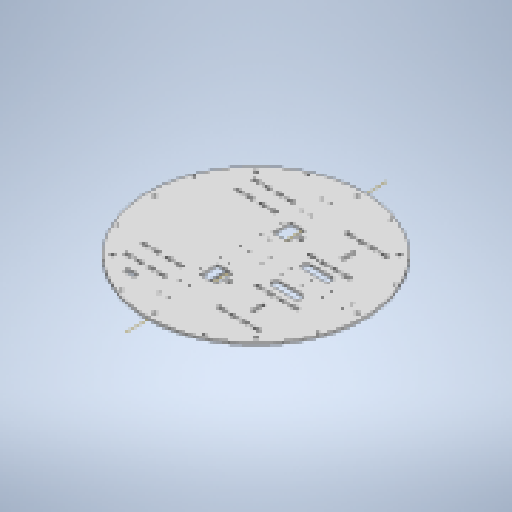
# Autodesk Inventor part: Osn. platform
Saved by Autodesk Inventor 2023.1 (Build 271208000, 208)
## iProperties
Created: 2023-03-13
Part Number: Osn. platform
Material: Типовые
Document SubType Name: Modeling
Designer: User
Density: 1 g/cm^3
Appearance: По умолчанию
Mass: 865.132 g
Surface Area: 3668.91 cm^2
Volume: 865.132 cm^3
Author: User
Autodesk Inventor part; units mm, degrees
ref_plane "YZ Plane" through (0, 0, 0) normal (1, 0, 0) x (0, 1, 0)
ref_plane "XZ Plane" through (0, 0, 0) normal (0, 1, 0) x (-1, 0, 0)
ref_plane "XY Plane" through (0, 0, 0) normal (0, 0, 1) x (1, 0, 0)
sketch "Основ. платформа" plane through (0, 0, 0) normal (0, 1, 0) x (-1, 0, 0)
  circle A0 centre (0, 0) radius 240
  line L0 (160.351, 321.3144) -> (160.351, -249.4153)
  point P0 (160.351, -178.5709)
  point P1 (160.351, 178.5709)
  dimension "d117" = 480
  constraints: 2 end point, 1 centre point, 1 coincident, 1 vertical
  measures "d117" diameter of A0
extrude "Осн. платформа" add sketch "Основ. платформа" along normal blind 5 contours L0 A0 picked at (27.6333, -10.8021)
sketch "Эскиз14" plane through (0, 5, 0) normal (0, 1, 0) x (0, 0, -1)
  line L0 (111.049, 144.9298) -> (124.3347, 144.9298)
  line L1 (124.3347, 144.9298) -> (124.3347, 138.9298)
  line L2 (111.049, 138.9298) -> (124.3347, 138.9298)
  line L3 (111.049, 144.9298) -> (111.049, 138.9298)
  line L4 (137.6204, 144.9298) -> (150.9061, 144.9298)
  line L5 (150.9061, 144.9298) -> (150.9061, 138.9298)
  line L6 (137.6204, 138.9298) -> (150.9061, 138.9298)
  line L7 (137.6204, 144.9298) -> (137.6204, 138.9298)
  line L8 (137.6204, 138.9298) -> (124.3347, 144.9298) construction
  line L9 (111.049, -61.9298) -> (124.3347, -61.9298)
  line L10 (111.049, -61.9298) -> (111.049, -55.9298)
  line L11 (97.7633, -61.9298) -> (97.7633, -55.9298)
  line L12 (71.1919, -61.9298) -> (71.1919, -55.9298)
  line L13 (57.9061, -61.9298) -> (57.9061, -55.9298)
  line L14 (57.9061, -55.9298) -> (71.1919, -55.9298)
  line L15 (57.9061, -61.9298) -> (71.1919, -61.9298)
  line L16 (107.4061, -87.5965) -> (101.4061, -87.5965)
  line L17 (101.4061, -87.5965) -> (101.4061, -113.2631)
  line L18 (107.4061, -113.2631) -> (107.4061, -87.5965)
  line L19 (57.9061, -138.9298) -> (71.1919, -138.9298)
  line L20 (101.4061, -113.2631) -> (107.4061, -113.2631)
  line L21 (84.4776, -138.9298) -> (97.7633, -138.9298)
  line L22 (84.4776, -144.9298) -> (84.4776, -138.9298)
  line L23 (84.4776, -144.9298) -> (97.7633, -144.9298)
  line L24 (97.7633, -144.9298) -> (97.7633, -138.9298)
  line L25 (111.049, -144.9298) -> (111.049, -138.9298)
  line L26 (111.049, -138.9298) -> (124.3347, -138.9298)
  line L27 (111.049, -144.9298) -> (124.3347, -144.9298)
  line L28 (124.3347, -144.9298) -> (124.3347, -138.9298)
  line L29 (137.6204, -61.9298) -> (150.9061, -61.9298)
  line L30 (150.9061, -61.9298) -> (150.9061, -55.9298)
  line L31 (137.6204, -55.9298) -> (150.9061, -55.9298)
  line L32 (137.6204, -61.9298) -> (137.6204, -55.9298)
  circle A0 centre (130.9776, -58.9298) radius 1.5
  line L33 (137.6204, -144.9298) -> (137.6204, -138.9298)
  line L34 (137.6204, -144.9298) -> (150.9061, -144.9298)
  line L35 (150.9061, -144.9298) -> (150.9061, -138.9298)
  line L36 (137.6204, -138.9298) -> (150.9061, -138.9298)
  line L37 (124.3347, -61.9298) -> (124.3347, -55.9298)
  line L38 (111.049, -55.9298) -> (124.3347, -55.9298)
  line L39 (84.4776, -61.9298) -> (97.7633, -61.9298)
  line L40 (84.4776, -55.9298) -> (97.7633, -55.9298)
  line L41 (84.4776, -61.9298) -> (84.4776, -55.9298)
  line L42 (71.1919, -144.9298) -> (71.1919, -138.9298)
  line L43 (57.9061, -144.9298) -> (71.1919, -144.9298)
  line L44 (57.9061, -144.9298) -> (57.9061, -138.9298)
  circle A1 centre (77.5336, -58.9298) radius 1.5
  circle A2 centre (130.9776, -141.9298) radius 1.5
  line L45 (137.6204, -138.9298) -> (124.3347, -144.9298) construction
  circle A3 centre (104.2556, -141.9298) radius 1.5
  circle A4 centre (77.5336, -141.9298) radius 1.5
  circle A5 centre (104.2556, -58.9298) radius 1.5
  line L46 (0, 238.0276) -> (0, -238.2088) construction
  line L47 (-70.7885, 145.0999) -> (-57.9314, 145.0999)
  line L48 (-57.9314, 145.0999) -> (-57.9314, 139.0999)
  line L49 (-57.9314, 139.0999) -> (-70.7885, 139.0999)
  line L50 (-70.7885, 139.0999) -> (-70.7885, 145.0999)
  line L51 (-70.7885, 106.8999) -> (-57.9314, 106.8999)
  line L52 (-57.9314, 106.8999) -> (-57.9314, 100.8999)
  line L53 (-57.9314, 100.8999) -> (-70.7885, 100.8999)
  line L54 (-70.7885, 100.8999) -> (-70.7885, 106.8999)
  line L55 (-70.7885, 145.0999) -> (-70.7885, 156.3999) construction
  line L56 (-70.7885, 100.8999) -> (-70.7885, 89.5999) construction
  line L57 (-96.5028, 100.8999) -> (-96.5028, 106.8999)
  line L58 (-96.5028, 106.8999) -> (-83.6457, 106.8999)
  line L59 (-83.6457, 139.0999) -> (-96.5028, 139.0999)
  line L60 (-83.6457, 100.8999) -> (-96.5028, 100.8999)
  line L61 (-83.6457, 145.0999) -> (-83.6457, 139.0999)
  line L62 (-96.5028, 139.0999) -> (-96.5028, 145.0999)
  line L63 (-96.5028, 145.0999) -> (-83.6457, 145.0999)
  line L64 (-83.6457, 106.8999) -> (-83.6457, 100.8999)
  line L65 (-122.2171, 100.8999) -> (-122.2171, 106.8999)
  line L66 (-122.2171, 106.8999) -> (-109.36, 106.8999)
  line L67 (-109.36, 139.0999) -> (-122.2171, 139.0999)
  line L68 (-109.36, 100.8999) -> (-122.2171, 100.8999)
  line L69 (-109.36, 145.0999) -> (-109.36, 139.0999)
  line L70 (-122.2171, 139.0999) -> (-122.2171, 145.0999)
  line L71 (-122.2171, 145.0999) -> (-109.36, 145.0999)
  line L72 (-109.36, 106.8999) -> (-109.36, 100.8999)
  line L73 (-147.9314, 100.8999) -> (-147.9314, 106.8999)
  line L74 (-147.9314, 106.8999) -> (-135.0743, 106.8999)
  line L75 (-135.0743, 139.0999) -> (-147.9314, 139.0999)
  line L76 (-135.0743, 100.8999) -> (-147.9314, 100.8999)
  line L77 (-135.0743, 145.0999) -> (-135.0743, 139.0999)
  line L78 (-147.9314, 139.0999) -> (-147.9314, 145.0999)
  line L79 (-147.9314, 145.0999) -> (-135.0743, 145.0999)
  line L80 (-135.0743, 106.8999) -> (-135.0743, 100.8999)
  line L81 (-135.0743, 139.0999) -> (-122.2171, 145.0999) construction
  line L82 (-83.6457, 139.0999) -> (-70.7885, 145.0999) construction
  line L83 (-135.0743, 100.8999) -> (-122.2171, 106.8999) construction
  line L84 (-83.6457, 100.8999) -> (-70.7885, 106.8999) construction
  circle A6 centre (-128.6457, 142.0999) radius 1.5
  circle A7 centre (-77.2171, 142.0999) radius 1.5
  circle A8 centre (-77.2171, 103.8999) radius 1.5
  circle A9 centre (-128.6457, 103.8999) radius 1.5
  line L85 (-147.9314, 145.0999) -> (-147.9314, 139.0999) projected
  line L86 (-135.0743, 145.0999) -> (-147.9314, 145.0999) projected
  arc A10 (-178.5709, 160.351) -> (178.5709, 160.351) centre (0, 0) ccw projected
  line L87 (-240, 0) -> (0, 0) construction
  line L88 (-122.2171, -139.0999) -> (-122.2171, -145.0999)
  line L89 (-147.9314, -145.0999) -> (-135.0743, -145.0999)
  line L90 (-147.9314, -139.0999) -> (-147.9314, -145.0999)
  line L91 (-96.5028, -106.8999) -> (-83.6457, -106.8999)
  line L92 (-96.5028, -100.8999) -> (-96.5028, -106.8999)
  line L93 (-83.6457, -100.8999) -> (-96.5028, -100.8999)
  line L94 (-83.6457, -106.8999) -> (-83.6457, -100.8999)
  line L95 (-83.6457, -100.8999) -> (-70.7885, -106.8999) construction
  circle A11 centre (-77.2171, -103.8999) radius 1.5
  line L96 (-70.7885, -100.8999) -> (-70.7885, -106.8999)
  line L97 (-70.7885, -106.8999) -> (-57.9314, -106.8999)
  line L98 (-57.9314, -106.8999) -> (-57.9314, -100.8999)
  line L99 (-57.9314, -100.8999) -> (-70.7885, -100.8999)
  line L100 (-70.7885, -100.8999) -> (-70.7885, -89.5999) construction
  line L101 (-122.2171, -100.8999) -> (-122.2171, -106.8999)
  line L102 (-147.9314, -100.8999) -> (-147.9314, -106.8999)
  line L103 (-135.0743, -145.0999) -> (-135.0743, -139.0999)
  line L104 (-135.0743, -139.0999) -> (-147.9314, -139.0999)
  line L105 (-147.9314, -106.8999) -> (-135.0743, -106.8999)
  line L106 (-135.0743, -106.8999) -> (-135.0743, -100.8999)
  line L107 (-135.0743, -100.8999) -> (-147.9314, -100.8999)
  line L108 (-109.36, -106.8999) -> (-109.36, -100.8999)
  line L109 (-109.36, -100.8999) -> (-122.2171, -100.8999)
  line L110 (-122.2171, -145.0999) -> (-109.36, -145.0999)
  line L111 (-122.2171, -106.8999) -> (-109.36, -106.8999)
  line L112 (-109.36, -139.0999) -> (-122.2171, -139.0999)
  circle A12 centre (-128.6457, -142.0999) radius 1.5
  circle A13 centre (-128.6457, -103.8999) radius 1.5
  line L113 (-135.0743, -100.8999) -> (-122.2171, -106.8999) construction
  line L114 (-109.36, -145.0999) -> (-109.36, -139.0999)
  line L115 (-135.0743, -139.0999) -> (-122.2171, -145.0999) construction
  line L116 (-70.7885, -145.0999) -> (-57.9314, -145.0999)
  line L117 (-57.9314, -145.0999) -> (-57.9314, -139.0999)
  line L118 (-57.9314, -139.0999) -> (-70.7885, -139.0999)
  line L119 (-70.7885, -139.0999) -> (-70.7885, -145.0999)
  circle A14 centre (-77.2171, -142.0999) radius 1.5
  line L120 (-83.6457, -139.0999) -> (-70.7885, -145.0999) construction
  line L121 (-83.6457, -145.0999) -> (-83.6457, -139.0999)
  line L122 (-70.7885, -145.0999) -> (-70.7885, -156.3999) construction
  line L123 (-96.5028, -145.0999) -> (-83.6457, -145.0999)
  line L124 (-96.5028, -139.0999) -> (-96.5028, -145.0999)
  line L125 (-83.6457, -139.0999) -> (-96.5028, -139.0999)
  line L126 (-147.9314, -145.0999) -> (-147.9314, -139.0999)
  line L127 (-135.0743, -145.0999) -> (-147.9314, -145.0999)
  line L128 (137.6204, 0) -> (-122.2171, 0) construction
  line L129 (97.7633, 61.9298) -> (97.7633, 55.9298)
  line L130 (84.4776, 55.9298) -> (97.7633, 55.9298)
  line L131 (84.4776, 61.9298) -> (84.4776, 55.9298)
  circle A15 centre (77.5336, 58.9298) radius 1.5
  line L132 (84.4776, 61.9298) -> (97.7633, 61.9298)
  circle A16 centre (104.2556, 58.9298) radius 1.5
  line L133 (111.049, 61.9298) -> (111.049, 55.9298)
  line L134 (111.049, 55.9298) -> (124.3347, 55.9298)
  line L135 (111.049, 61.9298) -> (124.3347, 61.9298)
  line L136 (124.3347, 61.9298) -> (124.3347, 55.9298)
  circle A17 centre (130.9776, 58.9298) radius 1.5
  line L137 (111.049, 138.9298) -> (124.3347, 138.9298)
  line L138 (111.049, 144.9298) -> (124.3347, 144.9298)
  line L139 (124.3347, 144.9298) -> (124.3347, 138.9298)
  circle A18 centre (130.9776, 141.9298) radius 1.5
  line L140 (137.6204, 138.9298) -> (124.3347, 144.9298) construction
  line L141 (137.6204, 144.9298) -> (137.6204, 138.9298)
  line L142 (137.6204, 138.9298) -> (150.9061, 138.9298)
  line L143 (137.6204, 144.9298) -> (150.9061, 144.9298)
  line L144 (150.9061, 144.9298) -> (150.9061, 138.9298)
  line L145 (137.6204, 61.9298) -> (137.6204, 55.9298)
  line L146 (137.6204, 55.9298) -> (150.9061, 55.9298)
  line L147 (137.6204, 61.9298) -> (150.9061, 61.9298)
  line L148 (150.9061, 61.9298) -> (150.9061, 55.9298)
  line L149 (107.4061, 87.5965) -> (101.4061, 87.5965)
  line L150 (101.4061, 87.5965) -> (101.4061, 113.2631)
  line L151 (107.4061, 113.2631) -> (107.4061, 87.5965)
  line L152 (111.049, 144.9298) -> (111.049, 138.9298)
  circle A19 centre (104.2556, 141.9298) radius 1.5
  line L153 (101.4061, 113.2631) -> (107.4061, 113.2631)
  line L154 (97.7633, 144.9298) -> (97.7633, 138.9298)
  line L155 (84.4776, 144.9298) -> (97.7633, 144.9298)
  line L156 (84.4776, 138.9298) -> (97.7633, 138.9298)
  line L157 (84.4776, 144.9298) -> (84.4776, 138.9298)
  circle A20 centre (77.5336, 141.9298) radius 1.5
  line L158 (71.1919, 61.9298) -> (71.1919, 55.9298)
  line L159 (57.9061, 144.9298) -> (57.9061, 138.9298)
  line L160 (57.9061, 144.9298) -> (71.1919, 144.9298)
  line L161 (71.1919, 144.9298) -> (71.1919, 138.9298)
  line L162 (57.9061, 138.9298) -> (71.1919, 138.9298)
  line L163 (57.9061, 61.9298) -> (57.9061, 55.9298)
  line L164 (57.9061, 61.9298) -> (71.1919, 61.9298)
  line L165 (57.9061, 55.9298) -> (71.1919, 55.9298)
  line L166 (11.3275, -97.2298) -> (11.3275, -64.2298) projected
  circle A21 centre (21.3275, -80.7298) radius 5.5
  circle A22 centre (19.3709, 80.7298) radius 5.5
  line L167 (9.3709, 64.2298) -> (9.3709, 97.2298) projected
  line L168 (11.3275, -80.7298) -> (40.4372, -80.7298)
  line L169 (9.3709, 80.7298) -> (30.4216, 80.7298)
  point P0 (-147.9314, -145.0886)
  point P1 (-147.9314, -145.0999)
  point P2 (-147.9108, -145.0999)
  point P3 (-135.0743, -145.0999)
  point P4 (-135.0743, 145.0999)
  point P5 (-147.9108, 145.0999)
  point P6 (-147.9314, 145.0999)
  point P7 (-147.9314, 145.0886)
  point P8 (-147.9314, 145.0999)
  dimension "d205" = 12.8571
  dimension "d206" = 6
  dimension "d207" = 25.7143
  dimension "d208" = 3
  dimension "d299" = 11
  dimension "d300" = 11
  dimension "d301" = 10
  dimension "d302" = 10
  constraints: 332 end point, 83 symmetric about line, 22 centre point, 8 equal length, 6 midpoint, 5 horizontal, 5 point on line, 3 equal radius, 2 collinear, 2 perpendicular, 2 vertical alignment, 1 point on circle, 1 vertical, 10 other
  measures "d205" distance of L48.end L49.end
  measures "d206" distance of L49.end L47.start
  measures "d207" distance of L54.start L57.start
  measures "d208" diameter of A9
  measures "d299" diameter of A21
  measures "d300" diameter of A22
  measures "d301" distance from line of L166 A21.centre
  measures "d302" distance from line of L167 A22.centre
extrude "Выдавливание9" cut sketch "Эскиз14" against normal up to surface (5 mm away)
sketch "Эскиз16" plane through (0, 5, 0) normal (0, 1, 0) x (0, 0, -1)
  line L0 (66.5859, 0) -> (-61.9521, 0) construction
  circle A0 centre (104.2556, -58.9298) radius 1.5 construction
  circle A1 centre (130.9776, -58.9298) radius 1.5 construction
  line L1 (125.6303, -33.4298) -> (77.5364, -33.4298) construction
  line L2 (125.6303, -24.4298) -> (77.5364, -24.4298)
  line L3 (77.5364, -42.4298) -> (125.6303, -42.4298)
  arc A2 (125.6303, -42.4298) -> (125.6303, -24.4298) centre (125.6303, -33.4298) ccw
  arc A3 (77.5364, -24.4298) -> (77.5364, -42.4298) centre (77.5364, -33.4298) ccw
  line L4 (125.6303, 33.4298) -> (77.5364, 33.4298) construction
  line L5 (125.6303, 24.4298) -> (77.5364, 24.4298)
  line L6 (77.5364, 42.4298) -> (125.6303, 42.4298)
  arc A4 (125.6303, 24.4298) -> (125.6303, 42.4298) centre (125.6303, 33.4298) ccw
  arc A5 (77.5364, 42.4298) -> (77.5364, 24.4298) centre (77.5364, 33.4298) ccw
  circle A6 centre (-225.3213, 0) radius 4
  circle A7 centre (-159.3262, -159.3262) radius 4
  circle A8 centre (0, -225.3213) radius 4
  circle A9 centre (159.3262, -159.3262) radius 4
  circle A10 centre (225.3213, 0) radius 4
  circle A11 centre (159.3262, 159.3262) radius 4
  circle A12 centre (0, 225.3213) radius 4
  circle A13 centre (-159.3262, 159.3262) radius 4
  line L7 (-57.9314, 100.8999) -> (-57.9314, 106.8999)
  line L8 (-70.7885, 100.8999) -> (-57.9314, 100.8999)
  line L9 (-70.9595, 100.7298) -> (-1.8725, 100.7298) construction
  line L10 (-70.9595, 100.7298) -> (-1.8725, 100.7298) construction
  line L11 (-23.8725, 60.7298) -> (-1.8725, 60.7298)
  line L12 (-1.8725, 60.7298) -> (-1.8725, 100.7298)
  line L13 (-1.8725, 100.7298) -> (-23.8725, 100.7298)
  line L14 (-23.8725, 100.7298) -> (-23.8725, 60.7298)
  line L15 (-23.8725, -60.7298) -> (-1.8725, -60.7298)
  line L16 (-1.8725, -60.7298) -> (-1.8725, -100.7298)
  line L17 (-1.8725, -100.7298) -> (-23.8725, -100.7298)
  line L18 (-23.8725, -100.7298) -> (-23.8725, -60.7298)
  circle A14 centre (104.2556, -141.9298) radius 1.5 construction
  line L19 (71.1919, -138.9298) -> (71.1919, -144.9298) construction
  line L20 (71.1919, -144.9298) -> (57.9061, -144.9298) construction
  line L21 (57.9061, -144.9298) -> (57.9061, -138.9298) construction
  line L22 (57.9061, -138.9298) -> (71.1919, -138.9298) construction
  line L23 (97.7633, -55.9298) -> (97.7633, -61.9298) construction
  line L24 (97.7633, -61.9298) -> (84.4776, -61.9298) construction
  line L25 (84.4776, -61.9298) -> (84.4776, -55.9298) construction
  line L26 (84.4776, -55.9298) -> (97.7633, -55.9298) construction
  circle A15 centre (77.5336, -58.9298) radius 1.5 construction
  line L27 (101.4061, -113.2631) -> (101.4061, -87.5965) construction
  line L28 (101.4061, -87.5965) -> (107.4061, -87.5965) construction
  line L29 (107.4061, -87.5965) -> (107.4061, -113.2631) construction
  line L30 (107.4061, -113.2631) -> (101.4061, -113.2631) construction
  line L31 (150.9061, -55.9298) -> (150.9061, -61.9298) construction
  line L32 (150.9061, -61.9298) -> (137.6204, -61.9298) construction
  line L33 (137.6204, -61.9298) -> (137.6204, -55.9298) construction
  line L34 (137.6204, -55.9298) -> (150.9061, -55.9298) construction
  circle A16 centre (104.2556, -58.9298) radius 1.5 construction
  circle A17 centre (130.9776, -141.9298) radius 1.5 construction
  circle A18 centre (77.5336, -141.9298) radius 1.5 construction
  line L35 (124.3347, -55.9298) -> (124.3347, -61.9298) construction
  line L36 (124.3347, -61.9298) -> (111.049, -61.9298) construction
  line L37 (111.049, -61.9298) -> (111.049, -55.9298) construction
  line L38 (111.049, -55.9298) -> (124.3347, -55.9298) construction
  line L39 (124.3347, -138.9298) -> (124.3347, -144.9298) construction
  line L40 (124.3347, -144.9298) -> (111.049, -144.9298) construction
  line L41 (111.049, -144.9298) -> (111.049, -138.9298) construction
  line L42 (111.049, -138.9298) -> (124.3347, -138.9298) construction
  line L43 (97.7633, -144.9298) -> (84.4776, -144.9298) construction
  line L44 (84.4776, -144.9298) -> (84.4776, -138.9298) construction
  line L45 (84.4776, -138.9298) -> (97.7633, -138.9298) construction
  line L46 (97.7633, -138.9298) -> (97.7633, -144.9298) construction
  line L47 (71.1919, -61.9298) -> (57.9061, -61.9298) construction
  line L48 (57.9061, -61.9298) -> (57.9061, -55.9298) construction
  line L49 (57.9061, -55.9298) -> (71.1919, -55.9298) construction
  line L50 (71.1919, -55.9298) -> (71.1919, -61.9298) construction
  line L51 (137.6204, -138.9298) -> (150.9061, -138.9298) construction
  line L52 (150.9061, -138.9298) -> (150.9061, -144.9298) construction
  line L53 (150.9061, -144.9298) -> (137.6204, -144.9298) construction
  line L54 (137.6204, -144.9298) -> (137.6204, -138.9298) construction
  circle A19 centre (130.9776, -58.9298) radius 1.5 construction
  arc A20 (-178.5709, 160.351) -> (178.5709, 160.351) centre (0, 0) ccw construction
  line L55 (-95.6688, -175.6959) -> (-112.4368, -171.5039) construction
  line L56 (-95.0528, -178.5999) -> (-113.0528, -178.5999)
  line L57 (-115.0528, -176.5999) -> (-115.0528, -170.5999)
  line L58 (-113.0528, -168.5999) -> (-95.0528, -168.5999)
  line L59 (-93.0528, -170.5999) -> (-93.0528, -176.5999)
  line L60 (-93.0528, -178.5999) -> (-115.0528, -168.5999) construction
  line L61 (-115.0528, -178.5999) -> (-93.0528, -168.5999) construction
  arc A21 (-113.0528, -168.5999) -> (-115.0528, -170.5999) centre (-113.0528, -170.5999) ccw
  arc A22 (-115.0528, -176.5999) -> (-113.0528, -178.5999) centre (-113.0528, -176.5999) ccw
  arc A23 (-95.0528, -178.5999) -> (-93.0528, -176.5999) centre (-95.0528, -176.5999) ccw
  arc A24 (-93.0528, -170.5999) -> (-95.0528, -168.5999) centre (-95.0528, -170.5999) ccw
  line L62 (-95.0509, -171.5999) -> (-95.0509, -175.5999) construction
  line L63 (-95.0509, -175.5999) -> (-113.0547, -175.5999) construction
  line L64 (-113.0547, -175.5999) -> (-113.0547, -171.5999) construction
  line L65 (-113.0547, -171.5999) -> (-95.0509, -171.5999) construction
  line L66 (-113.0547, -175.5999) -> (-95.0509, -171.5999) construction
  line L67 (-0.6725, -94.6798) -> (-0.6725, -99.2298)
  line L68 (-0.6725, -62.2298) -> (-0.6725, -66.7798)
  line L69 (-0.6725, -99.2298) -> (11.3275, -99.2298)
  line L70 (11.3275, -99.2298) -> (11.3275, -62.2298)
  line L71 (11.3275, -62.2298) -> (-0.6725, -62.2298)
  line L72 (-0.6725, -62.2298) -> (-0.6725, -99.2298)
  line L73 (-1.8725, 66.7798) -> (-1.8725, 62.2298)
  line L74 (-1.8725, 99.2298) -> (-1.8725, 94.6798)
  line L75 (-2.6291, 62.2298) -> (9.3709, 62.2298)
  line L76 (9.3709, 62.2298) -> (9.3709, 99.2298)
  line L77 (9.3709, 99.2298) -> (-2.6291, 99.2298)
  line L78 (-2.6291, 99.2298) -> (-2.6291, 62.2298)
  line L79 (-159.3262, -159.3262) -> (-225.3213, 0) construction
  line L80 (0, 0) -> (-272.8917, -124.0417) construction
  circle A25 centre (-211.5496, -96.1589) radius 2.5
  circle A26 centre (-81.5935, -217.5828) radius 2.5
  circle A27 centre (96.1589, -211.5496) radius 2.5
  circle A28 centre (217.5828, -81.5935) radius 2.5
  circle A29 centre (211.5496, 96.1589) radius 2.5
  circle A30 centre (81.5935, 217.5828) radius 2.5
  circle A31 centre (-96.1589, 211.5496) radius 2.5
  circle A32 centre (-217.5828, 81.5935) radius 2.5
  line L81 (178.5709, 160.351) -> (-178.5709, 160.351)
  point P0 (101.5834, -33.4298)
  point P1 (101.5834, 33.4298)
  point P2 (-104.0528, -173.5999)
  point P3 (-1.8725, -62.2298)
  point P4 (-1.8725, -99.2298)
extrude "Выдавливание10" cut sketch "Эскиз16" against normal blind 10 contours A2 L3 A3 L2 | L5 A5 L6 A4 | A6 | A7 | A8 | A9 | A10 | A12 | L14 L13 L12 L77 L78 L75 L11 | L75 L78 L77 L12 | L12 L77 L76 L75 | L15 L16 L17 L18 | L56 A22 L57 A21 L58 A24 L59 A23 | L72 L68 L71 L70 L69 L67 | A25 | A26 | A27 | A28 | A29 | A30 | A31 | A32
sketch "Эскиз22" plane through (0, 0, 0) normal (0, -1, 0) x (0, 0, -1)
  line L0 (-43.8725, 199.9715) -> (-36.9425, 199.9715) construction
  line L1 (-36.9425, 199.9715) -> (-36.9425, -200.0285) construction
  line L2 (-36.9425, -200.0285) -> (-43.8725, -200.0285) construction
  line L3 (-43.8725, -200.0285) -> (-43.8725, 199.9715) construction
  line L4 (-30.8025, 199.9715) -> (-26.6225, 199.9715) construction
  line L5 (-26.6225, 199.9715) -> (-24.9495, 199.9715) construction
  line L6 (-24.9495, 199.9715) -> (-22.7955, 199.9715) construction
  line L7 (-22.7955, 199.9715) -> (-21.1225, 199.9715) construction
  line L8 (-21.1225, 199.9715) -> (-16.9425, 199.9715) construction
  line L9 (-16.9425, 199.9715) -> (-16.9425, -200.0285) construction
  line L10 (-16.9425, -200.0285) -> (-21.1225, -200.0285) construction
  line L11 (-21.1225, -200.0285) -> (-21.1225, 199.9715) construction
  line L12 (-30.8025, -200.0285) -> (-30.8025, 199.9715) construction
  line L13 (-26.6225, -200.0285) -> (-30.8025, -200.0285) construction
  line L14 (-26.6225, -200.0285) -> (-26.6225, 199.9715) construction
  line L15 (-24.9495, 199.9715) -> (-24.9495, -200.0285) construction
  line L16 (-24.9495, -200.0285) -> (-26.6225, -200.0285) construction
  line L17 (-22.7955, 199.9715) -> (-22.7955, -200.0285) construction
  line L18 (-22.7955, -200.0285) -> (-24.9495, -200.0285) construction
  line L19 (-21.1225, -200.0285) -> (-22.7955, -200.0285) construction
  line L20 (-10.8025, 199.9715) -> (-3.8725, 199.9715) construction
  line L21 (-3.8725, 199.9715) -> (-3.8725, -200.0285) construction
  line L22 (-3.8725, -200.0285) -> (-10.8025, -200.0285) construction
  line L23 (-10.8025, -200.0285) -> (-10.8025, 199.9715) construction
  line L24 (-3.8725, -19.9998) -> (-3.8725, -15.4498) construction
  line L25 (226.1275, -15.4498) -> (-3.8725, -15.4498) construction
  line L26 (226.1275, -15.4498) -> (226.1275, -19.9998) construction
  line L27 (226.1275, -19.9998) -> (-3.8725, -19.9998) construction
  line L28 (-3.8725, -7.5498) -> (-3.8725, -1.9588) construction
  line L29 (226.1275, -1.9588) -> (-3.8725, -1.9588) construction
  line L30 (226.1275, -1.9588) -> (226.1275, -7.5498) construction
  line L31 (226.1275, -7.5498) -> (-3.8725, -7.5498) construction
  line L32 (-3.8725, -1.0408) -> (-3.8725, 4.5502) construction
  line L33 (226.1275, 4.5502) -> (-3.8725, 4.5502) construction
  line L34 (226.1275, 4.5502) -> (226.1275, -1.0408) construction
  line L35 (226.1275, -1.0408) -> (-3.8725, -1.0408) construction
  line L36 (-3.8725, 12.4502) -> (-3.8725, 17.0002) construction
  line L37 (226.1275, 17.0002) -> (-3.8725, 17.0002) construction
  line L38 (226.1275, 17.0002) -> (226.1275, 12.4502) construction
  line L39 (226.1275, 12.4502) -> (-3.8725, 12.4502) construction
  line L40 (-43.8725, 199.9715) -> (-36.9425, 199.9715) construction
  line L41 (-36.9425, 199.9715) -> (-36.9425, -200.0285) construction
  line L42 (-36.9425, -200.0285) -> (-43.8725, -200.0285) construction
  line L43 (-43.8725, -200.0285) -> (-43.8725, 199.9715) construction
  line L44 (-30.8025, 199.9715) -> (-26.6225, 199.9715) construction
  line L45 (-26.6225, 199.9715) -> (-24.9495, 199.9715) construction
  line L46 (-24.9495, 199.9715) -> (-22.7955, 199.9715) construction
  line L47 (-22.7955, 199.9715) -> (-21.1225, 199.9715) construction
  line L48 (-21.1225, 199.9715) -> (-16.9425, 199.9715) construction
  line L49 (-16.9425, 199.9715) -> (-16.9425, -200.0285) construction
  line L50 (-16.9425, -200.0285) -> (-21.1225, -200.0285) construction
  line L51 (-21.1225, -200.0285) -> (-21.1225, 199.9715) construction
  line L52 (-30.8025, -200.0285) -> (-30.8025, 199.9715) construction
  line L53 (-26.6225, -200.0285) -> (-30.8025, -200.0285) construction
  line L54 (-26.6225, -200.0285) -> (-26.6225, 199.9715) construction
  line L55 (-24.9495, 199.9715) -> (-24.9495, -200.0285) construction
  line L56 (-24.9495, -200.0285) -> (-26.6225, -200.0285) construction
  line L57 (-22.7955, 199.9715) -> (-22.7955, -200.0285) construction
  line L58 (-22.7955, -200.0285) -> (-24.9495, -200.0285) construction
  line L59 (-21.1225, -200.0285) -> (-22.7955, -200.0285) construction
  line L60 (-10.8025, 199.9715) -> (-3.8725, 199.9715) construction
  line L61 (-3.8725, 199.9715) -> (-3.8725, -200.0285) construction
  line L62 (-3.8725, -200.0285) -> (-10.8025, -200.0285) construction
  line L63 (-10.8025, -200.0285) -> (-10.8025, 199.9715) construction
  line L64 (-43.8725, 199.9715) -> (-36.9425, 199.9715) construction
  line L65 (-36.9425, 199.9715) -> (-36.9425, -200.0285) construction
  line L66 (-36.9425, -200.0285) -> (-43.8725, -200.0285) construction
  line L67 (-43.8725, -200.0285) -> (-43.8725, 199.9715) construction
  line L68 (-30.8025, 199.9715) -> (-26.6225, 199.9715) construction
  line L69 (-26.6225, 199.9715) -> (-24.9495, 199.9715) construction
  line L70 (-24.9495, 199.9715) -> (-22.7955, 199.9715) construction
  line L71 (-22.7955, 199.9715) -> (-21.1225, 199.9715) construction
  line L72 (-21.1225, 199.9715) -> (-16.9425, 199.9715) construction
  line L73 (-16.9425, 199.9715) -> (-16.9425, -200.0285) construction
  line L74 (-16.9425, -200.0285) -> (-21.1225, -200.0285) construction
  line L75 (-21.1225, -200.0285) -> (-21.1225, 199.9715) construction
  line L76 (-30.8025, -200.0285) -> (-30.8025, 199.9715) construction
  line L77 (-26.6225, -200.0285) -> (-30.8025, -200.0285) construction
  line L78 (-26.6225, -200.0285) -> (-26.6225, 199.9715) construction
  line L79 (-24.9495, 199.9715) -> (-24.9495, -200.0285) construction
  line L80 (-24.9495, -200.0285) -> (-26.6225, -200.0285) construction
  line L81 (-22.7955, 199.9715) -> (-22.7955, -200.0285) construction
  line L82 (-22.7955, -200.0285) -> (-24.9495, -200.0285) construction
  line L83 (-21.1225, -200.0285) -> (-22.7955, -200.0285) construction
  line L84 (-10.8025, 199.9715) -> (-3.8725, 199.9715) construction
  line L85 (-3.8725, 199.9715) -> (-3.8725, -200.0285) construction
  line L86 (-3.8725, -200.0285) -> (-10.8025, -200.0285) construction
  line L87 (-10.8025, -200.0285) -> (-10.8025, 199.9715) construction
  line L88 (-16.9425, 199.9715) -> (-10.8025, 199.9715) construction
  line L89 (-10.8025, 199.9715) -> (-10.8025, -200.0285) construction
  line L90 (-10.8025, -200.0285) -> (-16.9425, -200.0285) construction
  line L91 (-16.9425, -200.0285) -> (-16.9425, 199.9715) construction
  line L92 (-16.9425, -200.0285) -> (-10.8025, 199.9715) construction
  line L93 (-16.9425, 199.9715) -> (-10.8025, -200.0285)
  circle A0 centre (-13.8725, -0.0285) radius 1.575
  circle A1 centre (-13.8725, 44.9715) radius 1.575
  circle A2 centre (-13.8725, 89.9715) radius 1.575
  circle A3 centre (-13.8725, 134.9715) radius 1.575
  circle A4 centre (-13.8725, 179.9715) radius 1.575
  line L94 (-30.8025, -199.8158) -> (-36.9425, 199.9715)
  line L95 (-30.8025, 199.9715) -> (-36.9425, -200.0285) construction
  circle A5 centre (-33.8725, -0.0285) radius 1.575
  circle A6 centre (-13.8725, -45.0285) radius 1.575
  circle A7 centre (-33.8725, -45.0285) radius 1.575
  circle A8 centre (-13.8725, -90.0285) radius 1.575
  circle A9 centre (-33.8725, -90.0285) radius 1.575
  circle A10 centre (-13.8725, -135.0285) radius 1.575
  circle A11 centre (-33.8725, -135.0285) radius 1.575
  circle A12 centre (-13.8725, -180.0285) radius 1.575
  circle A13 centre (-33.8725, -180.0285) radius 1.575
  circle A14 centre (-33.8725, 44.9715) radius 1.575
  circle A15 centre (-33.8725, 89.9715) radius 1.575
  circle A16 centre (-33.8725, 134.9715) radius 1.575
  circle A17 centre (-33.8725, 179.9715) radius 1.575
  line L96 (226.1275, -7.5498) -> (-3.8725, -15.4498) construction
  line L97 (-3.8725, -7.5498) -> (226.1275, -15.4498)
  line L98 (226.1275, 12.4502) -> (-3.8725, 4.5502)
  line L99 (-3.8725, 12.4502) -> (226.1275, 4.5502) construction
  circle A18 centre (111.1275, 8.5002) radius 1.575
  line L100 (-36.9425, 179.9715) -> (-36.9425, -220.0285) construction
  circle A19 centre (111.1275, -11.4998) radius 1.575
  line L101 (-81.9425, 199.9715) -> (-81.9425, -200.0285) construction
  circle A20 centre (66.1275, 8.5002) radius 1.575
  line L102 (-81.9425, 179.9715) -> (-81.9425, -220.0285) construction
  circle A21 centre (66.1275, -11.4998) radius 1.575
  line L103 (-126.9425, 199.9715) -> (-126.9425, -200.0285) construction
  circle A22 centre (21.1275, 8.5002) radius 1.575
  line L104 (-126.9425, 179.9715) -> (-126.9425, -220.0285) construction
  circle A23 centre (21.1275, -11.4998) radius 1.575
  circle A24 centre (111.1275, -11.4998) radius 1.575
  circle A25 centre (156.1275, 8.5002) radius 1.575
  circle A26 centre (156.1275, -11.4998) radius 1.575
  circle A27 centre (201.1275, 8.5002) radius 1.575
  circle A28 centre (201.1275, -11.4998) radius 1.575
  point P0 (0, 0)
  point P1 (-33.8725, -0.0285)
  point P2 (-33.8725, 44.9715)
  point P3 (-33.8725, 89.9715)
  point P4 (-33.8725, 134.9715)
  point P5 (-33.8725, 179.9715)
  point P6 (111.1275, -11.4998)
  dimension "d250" = 3.15
  dimension "d260" = 45
  dimension "d267" = 20
  dimension "d270" = 45
  dimension "d275" = 45
  dimension "d280" = 3.15
  dimension "d283" = 20
  dimension "d286" = 45
  dimension "d291" = 20
  dimension "d294" = 45
  constraints: 204 end point, 49 horizontal, 40 vertical, 29 centre point, 4 midpoint, 2 parallel, 1 coincident, 1 perpendicular, 1 point on line, 123 other
  measures "d250" diameter of A0
  measures "d260" distance of A0.centre A1.centre
  measures "d267" distance of A0.centre A5.centre
  measures "d270" distance of A0.centre A6.centre
  measures "d275" distance of point (-33.872, -0.029) point (-33.872, 44.971)
  measures "d280" diameter of A18
  measures "d283" distance of L0.end L100.start
  measures "d286" distance of L0.end L101.start
  measures "d291" distance of A18.centre A24.centre
  measures "d294" distance of A18.centre A25.centre
extrude "Выдавливание13" cut sketch "Эскиз22" against normal blind 10 contours A1 L93 | L93 A1 | A0 L93 | L93 A0 | A6 L93 | L93 A6 | A8 L93 | L93 A8 | A3 | A4 | A9 L94 | L94 A9 | A7 L94 | L94 A7 | A5 L94 | L94 A5 | A14 L94 | L94 A14 | A15 L94 | L94 A15 | A10 | A11 | A12 | A13 | A16 | A17 | A21 L97 | L97 A21 | A19 L97 | L97 A19 | A26 L97 | L97 A26 | A25 L98 | L98 A25 | A18 L98 | L98 A18 | A20 L98 | L98 A20 | A22 | A23 | A27 | A28
